Autodesk Inventor part; units mm, degrees
(part 2 of 2)
sketch "Sketch29" plane through (0, 0, -31) normal (0, 0, -1) x (-1, 0, 0)
  line L0 (66.4684, -62.625) -> (66.4684, -59.625) projected
  line L1 (76.0516, -62.625) -> (66.4684, -62.625) projected
  line L2 (76.0516, -59.625) -> (76.0516, -62.625) projected
  line L3 (76.0516, -59.625) -> (66.4684, -59.625) projected
  line L4 (86.26, -59.625) -> (86.26, -56.625) projected
  line L5 (86.26, -56.625) -> (-49.26, -56.625) projected
  arc A0 (-54.26, -51.625) -> (-49.26, -56.625) centre (-49.26, -51.625) ccw projected
  line L6 (-54.26, -51.625) -> (-54.26, 34.625) projected
  line L7 (-54.26, 34.625) -> (-57.26, 34.625) projected
  line L8 (-57.26, 34.625) -> (-57.26, -51.625) projected
  arc A1 (-57.26, -51.625) -> (-49.26, -59.625) centre (-49.26, -51.625) ccw projected
  line L9 (-49.26, -59.625) -> (86.26, -59.625) projected
  line L10 (76.26, -60.625) -> (66.26, -60.625)
  line L11 (66.26, -60.625) -> (66.26, -52.625)
  line L12 (66.26, -52.625) -> (76.26, -52.625)
  line L13 (76.26, -52.625) -> (76.26, -60.625)
  line L14 (50.26, -56.625) -> (86.26, -56.625) projected
  line L15 (76.26, -60.625) -> (66.26, -52.625) construction
  line L16 (66.26, -60.625) -> (76.26, -52.625) construction
  point P0 (0, 0)
  point P1 (71.26, -56.625)
  point P2 (66.26, -56.625)
  point P3 (76.26, -56.625)
  dimension "d214" = 10
  dimension "d215" = 8
  constraints: 12 end point, 2 midpoint, 2 parallel, 1 horizontal, 1 perpendicular, 1 point on line
  measures "d214" distance of L11.end L12.end
  measures "d215" distance of L10.end L11.end
extrude "Extrusion21" add sketch "Sketch29" against normal blind 10 contours L11 L12 L13 L5
sketch "Sketch30" plane through (0, 0, -31) normal (0, 0, -1) x (-1, 0, 0)
  line L0 (86.26, -59.625) -> (86.26, -56.625) projected
  line L1 (86.26, -56.625) -> (76.26, -56.625) projected
  line L2 (76.26, -56.625) -> (76.26, -52.625) projected
  line L3 (76.26, -52.625) -> (66.26, -52.625) projected
  line L4 (66.26, -52.625) -> (66.26, -56.625) projected
  line L5 (66.26, -56.625) -> (-49.26, -56.625) projected
  arc A0 (-54.26, -51.625) -> (-49.26, -56.625) centre (-49.26, -51.625) ccw projected
  line L6 (-54.26, -51.625) -> (-54.26, 34.625) projected
  line L7 (-54.26, 34.625) -> (-57.26, 34.625) projected
  line L8 (-57.26, 34.625) -> (-57.26, -51.625) projected
  arc A1 (-57.26, -51.625) -> (-49.26, -59.625) centre (-49.26, -51.625) ccw projected
  line L9 (-49.26, -59.625) -> (86.26, -59.625) projected
  line L10 (66.26, -56.625) -> (76.26, -56.625)
  line L11 (66.26, -56.625) -> (76.26, -56.625) projected
  line L12 (68.46, -56.625) -> (74.06, -56.625)
  line L13 (74.06, -56.625) -> (74.06, -54.025)
  line L14 (74.06, -54.025) -> (68.46, -54.025)
  line L15 (68.46, -54.025) -> (68.46, -56.625)
  line L16 (76.26, -52.625) -> (66.26, -52.625) projected
  point P0 (0, 0)
  point P1 (71.26, -54.025)
  point P2 (71.26, -52.625)
  point P3 (71.26, -52.625)
  dimension "d218" = 5.6
  dimension "d219" = 2.6
  constraints: 10 end point, 3 midpoint, 2 horizontal, 2 parallel, 1 perpendicular, 1 point on line, 1 vertical alignment
  measures "d218" distance of L14.end L13.end
  measures "d219" distance of L13.end L12.end
extrude "Extrusion22" cut sketch "Sketch30" against normal blind 7 contours L10 L15 L14 L13
chamfer "Chamfer9" distance 2 angle 45 2 edges at (-71.26, -56.625, -21) (-71.26, -52.625, -21)
fillet "Fillet6" radius 3 4 edges at (-76.26, -56.625, -26) (-76.26, -56.625, -20.0001) (-66.26, -56.625, -26) (-66.26, -56.625, -20.0001)
sketch "Sketch31" plane through (0, 0, -31) normal (0, 0, -1) x (-1, 0, 0)
  line L0 (74.06, -56.625) -> (68.46, -56.625) projected
  line L1 (68.46, -56.625) -> (68.46, -54.025) projected
  line L2 (68.46, -54.025) -> (74.06, -54.025) projected
  line L3 (74.06, -54.025) -> (74.06, -56.625) projected
  line L4 (86.26, -59.625) -> (86.26, -56.625) projected
  line L5 (86.26, -56.625) -> (79.26, -56.625) projected
  arc A0 (76.26, -53.625) -> (79.26, -56.625) centre (79.26, -53.625) ccw projected
  line L6 (76.26, -53.625) -> (76.26, -52.625) projected
  line L7 (76.26, -52.625) -> (66.26, -52.625) projected
  line L8 (66.26, -52.625) -> (66.26, -53.625) projected
  arc A1 (63.26, -56.625) -> (66.26, -53.625) centre (63.26, -53.625) ccw projected
  line L9 (63.26, -56.625) -> (-49.26, -56.625) projected
  arc A2 (-54.26, -51.625) -> (-49.26, -56.625) centre (-49.26, -51.625) ccw projected
  line L10 (-54.26, -51.625) -> (-54.26, 34.625) projected
  line L11 (-54.26, 34.625) -> (-57.26, 34.625) projected
  line L12 (-57.26, 34.625) -> (-57.26, -51.625) projected
  arc A3 (-57.26, -51.625) -> (-49.26, -59.625) centre (-49.26, -51.625) ccw projected
  line L13 (-49.26, -59.625) -> (86.26, -59.625) projected
  line L14 (-57.26, -23.1666) -> (-60.26, -23.1666) projected
  line L15 (-57.26, -23.1666) -> (-57.26, -13.5834) projected
  line L16 (-60.26, -13.5834) -> (-57.26, -13.5834) projected
  line L17 (-60.26, -23.1666) -> (-60.26, -13.5834) projected
  line L18 (-58.26, -23.375) -> (-50.26, -23.375)
  line L19 (-50.26, -23.375) -> (-50.26, -13.375)
  line L20 (-50.26, -13.375) -> (-58.26, -13.375)
  line L21 (-58.26, -13.375) -> (-58.26, -23.375)
  line L22 (-54.26, 55.625) -> (-54.26, -51.625) projected
  line L23 (-58.26, -23.375) -> (-50.26, -13.375) construction
  line L24 (-50.26, -23.375) -> (-58.26, -13.375) construction
  point P0 (0, 0)
  point P1 (-54.26, -18.375)
  point P2 (-54.26, -13.375)
  point P3 (-54.26, -23.375)
  dimension "d226" = 8
  dimension "d227" = 10
  constraints: 12 end point, 2 midpoint, 2 parallel, 1 horizontal, 1 perpendicular, 1 point on line
  measures "d226" distance of L20.end L19.end
  measures "d227" distance of L19.end L18.end
extrude "Extrusion23" add sketch "Sketch31" against normal blind 10 contours L10 L20 L19 L18
sketch "Sketch26" plane through (57.26, -51.625, -31) normal (1, 0, 0) x (0, 0, -1)
  arc A0 (-4, 38.25) -> (-4, 28.25) centre (-4, 33.25) ccw projected
  point P0 (-31, 51.625)
hole "Hole6" at (57.26, -18.375, -27) direction (-1, 0, 0) diameter 3.4 depth 8 clearance for "Socket Head Cap Screw" size "M3" standard "Ansi Metric M Profile"
sketch "Sketch27" plane through (-86.26, -59.625, -31) normal (0, -1, 0) x (1, 0, 0)
  arc A0 (20, 4) -> (10, 4) centre (15, 4) ccw projected
  point P0 (86.26, 31)
hole "Hole7" at (-71.26, -59.625, -27) direction (0, 1, 0) diameter 3.4 depth 8 clearance for "Socket Head Cap Screw" size "M3" standard "Ansi Metric M Profile"
sketch "Sketch32" plane through (0, 0, -31) normal (0, 0, -1) x (-1, 0, 0)
  line L0 (74.06, -56.625) -> (68.46, -56.625) projected
  line L1 (68.46, -56.625) -> (68.46, -54.025) projected
  line L2 (68.46, -54.025) -> (74.06, -54.025) projected
  line L3 (74.06, -54.025) -> (74.06, -56.625) projected
  line L4 (86.26, -59.625) -> (86.26, -56.625) projected
  line L5 (86.26, -56.625) -> (79.26, -56.625) projected
  arc A0 (76.26, -53.625) -> (79.26, -56.625) centre (79.26, -53.625) ccw projected
  line L6 (76.26, -53.625) -> (76.26, -52.625) projected
  line L7 (76.26, -52.625) -> (66.26, -52.625) projected
  line L8 (66.26, -52.625) -> (66.26, -53.625) projected
  arc A1 (63.26, -56.625) -> (66.26, -53.625) centre (63.26, -53.625) ccw projected
  line L9 (63.26, -56.625) -> (-49.26, -56.625) projected
  arc A2 (-54.26, -51.625) -> (-49.26, -56.625) centre (-49.26, -51.625) ccw projected
  line L10 (-54.26, -51.625) -> (-54.26, -23.375) projected
  line L11 (-54.26, -23.375) -> (-50.26, -23.375) projected
  line L12 (-50.26, -23.375) -> (-50.26, -13.375) projected
  line L13 (-50.26, -13.375) -> (-54.26, -13.375) projected
  line L14 (-54.26, -13.375) -> (-54.26, 34.625) projected
  line L15 (-54.26, 34.625) -> (-57.26, 34.625) projected
  line L16 (-57.26, 34.625) -> (-57.26, -51.625) projected
  arc A3 (-57.26, -51.625) -> (-49.26, -59.625) centre (-49.26, -51.625) ccw projected
  line L17 (-49.26, -59.625) -> (86.26, -59.625) projected
  line L18 (-54.26, -51.625) -> (-54.26, -23.375) projected
  line L19 (-54.26, -13.375) -> (-54.26, -23.375)
  line L20 (-56.86, -21.175) -> (-51.66, -21.175)
  line L21 (-51.66, -21.175) -> (-51.66, -15.575)
  line L22 (-51.66, -15.575) -> (-56.86, -15.575)
  line L23 (-56.86, -15.575) -> (-56.86, -21.175)
  line L24 (-56.86, -21.175) -> (-51.66, -15.575) construction
  line L25 (-51.66, -21.175) -> (-56.86, -15.575) construction
  point P0 (0, 0)
  point P1 (-54.26, -18.375)
  point P2 (-54.26, -15.575)
  point P3 (-54.26, -21.175)
  dimension "d238" = 5.2
  dimension "d239" = 5.6
  constraints: 14 end point, 3 midpoint, 2 parallel, 1 horizontal, 1 perpendicular, 1 vertical
  measures "d238" distance of L22.end L21.end
  measures "d239" distance of L21.end L20.end
extrude "Extrusion24" cut sketch "Sketch32" against normal blind 7.5 contours L22 L21 L20 L19
chamfer "Chamfer10" distance 2 angle 45 2 edges at (50.26, -18.375, -21) (54.26, -18.375, -21)
fillet "Fillet7" radius 4 4 edges at (54.26, -23.375, -20.0001) (54.26, -23.375, -26) (54.26, -13.375, -20.0001) (54.26, -13.375, -26)
sketch "Sketch33" plane through (-86.26, -62.625, 5.75) normal (0, -1, 0) x (1, 0, 0)
  line L0 (115.9766, -20.7763) -> (-67.1269, -20.7763) construction
  line L1 (-67.1269, -20.7763) -> (-67.1269, -9.2572) construction
  line L2 (-67.1269, -9.2572) -> (115.9766, -9.2572) construction
  line L3 (115.9766, -9.2572) -> (115.9766, -20.7763) construction
  line L4 (115.1682, -20.6377) -> (111.0565, -20.6377)
  spline S0 degree 2 poles (111.0565, -20.6377) (109.7168, -20.6377) (108.377, -19.3595) (108.377, -18.1815) knots 0 0 0 1 2 2 2
  spline S1 degree 2 poles (108.377, -18.1815) (108.377, -16.9649) (109.8323, -15.6021) (111.326, -15.6021) knots 0 0 0 1 2 2 2
  line L5 (111.326, -15.6021) -> (112.6811, -15.6021)
  line L6 (112.6811, -15.6021) -> (112.6811, -12.6377)
  line L7 (112.6811, -12.6377) -> (115.1682, -12.6377)
  line L8 (115.1682, -12.6377) -> (115.1682, -20.6377)
  line L9 (112.6811, -17.2267) -> (112.0806, -17.2267)
  spline S2 degree 2 poles (112.0806, -17.2267) (111.3645, -17.2267) (110.787, -17.7272) (110.787, -18.1122) knots 0 0 0 1 2 2 2
  spline S3 degree 2 poles (110.787, -18.1122) (110.787, -18.4895) (111.2875, -19.0131) (111.9805, -19.0131) knots 0 0 0 1 2 2 2
  line L10 (111.9805, -19.0131) -> (112.6811, -19.0131)
  line L11 (112.6811, -19.0131) -> (112.6811, -17.2267)
  line L12 (107.0835, -20.6377) -> (100.4617, -20.6377)
  line L13 (100.4617, -20.6377) -> (100.4617, -18.9284)
  line L14 (100.4617, -18.9284) -> (104.6041, -18.9284)
  line L15 (104.6041, -18.9284) -> (104.6041, -17.6579)
  line L16 (104.6041, -17.6579) -> (100.762, -17.6579)
  line L17 (100.762, -17.6579) -> (100.762, -16.0256)
  line L18 (100.762, -16.0256) -> (104.6041, -16.0256)
  line L19 (104.6041, -16.0256) -> (104.6041, -14.4471)
  line L20 (104.6041, -14.4471) -> (100.3385, -14.4471)
  line L21 (100.3385, -14.4471) -> (100.3385, -12.6377)
  line L22 (100.3385, -12.6377) -> (107.0835, -12.6377)
  line L23 (107.0835, -12.6377) -> (107.0835, -20.6377)
  line L24 (99.0142, -20.6377) -> (94.9025, -20.6377)
  spline S4 degree 2 poles (94.9025, -20.6377) (93.5628, -20.6377) (92.223, -19.3595) (92.223, -18.1815) knots 0 0 0 1 2 2 2
  spline S5 degree 2 poles (92.223, -18.1815) (92.223, -16.9649) (93.6783, -15.6021) (95.172, -15.6021) knots 0 0 0 1 2 2 2
  line L25 (95.172, -15.6021) -> (96.5271, -15.6021)
  line L26 (96.5271, -15.6021) -> (96.5271, -12.6377)
  line L27 (96.5271, -12.6377) -> (99.0142, -12.6377)
  line L28 (99.0142, -12.6377) -> (99.0142, -20.6377)
  line L29 (96.5271, -17.2267) -> (95.9266, -17.2267)
  spline S6 degree 2 poles (95.9266, -17.2267) (95.2105, -17.2267) (94.633, -17.7272) (94.633, -18.1122) knots 0 0 0 1 2 2 2
  spline S7 degree 2 poles (94.633, -18.1122) (94.633, -18.4895) (95.1335, -19.0131) (95.8265, -19.0131) knots 0 0 0 1 2 2 2
  line L30 (95.8265, -19.0131) -> (96.5271, -19.0131)
  line L31 (96.5271, -19.0131) -> (96.5271, -17.2267)
  line L32 (81.8746, -15.9101) -> (79.711, -15.2556)
  spline S8 degree 2 poles (79.711, -15.2556) (79.9266, -14.347) (80.8659, -13.1228) (82.2596, -12.4991) (83.3298, -12.4991) knots 0 0 0 1 2 3 3 3
  spline S9 degree 2 poles (83.3298, -12.4991) (84.6388, -12.4991) (86.2865, -13.2614) (87.4877, -15.1709) (87.4877, -16.6569) knots 0 0 0 1 2 3 3 3
  spline S10 degree 2 poles (87.4877, -16.6569) (87.4877, -18.6435) (85.378, -20.7763) (83.4453, -20.7763) knots 0 0 0 1 2 2 2
  spline S11 degree 2 poles (83.4453, -20.7763) (81.9362, -20.7763) (80.2115, -19.552) (79.788, -18.2893) knots 0 0 0 1 2 2 2
  line L33 (79.788, -18.2893) -> (81.9747, -17.8042)
  spline S12 degree 2 poles (81.9747, -17.8042) (82.0902, -18.1661) (82.2134, -18.3355) knots 0 0 0 1 1 1
  spline S13 degree 2 poles (82.2134, -18.3355) (82.4213, -18.6204) (83.0219, -18.9284) (83.3914, -18.9284) knots 0 0 0 1 2 2 2
  spline S14 degree 2 poles (83.3914, -18.9284) (84.223, -18.9284) (84.6696, -18.2508) knots 0 0 0 1 1 1
  spline S15 degree 2 poles (84.6696, -18.2508) (85.0084, -17.7503) (85.0084, -16.6723) knots 0 0 0 1 1 1
  spline S16 degree 2 poles (85.0084, -16.6723) (85.0084, -15.3403) (84.1999, -14.3547) (83.4684, -14.3547) knots 0 0 0 1 2 2 2
  spline S17 degree 2 poles (83.4684, -14.3547) (82.7601, -14.3547) (82.0363, -15.1478) (81.8746, -15.9101) knots 0 0 0 1 2 2 2
  spline S18 degree 2 poles (78.8101, -16.6338) (78.8101, -18.5896) (76.6234, -20.7763) (74.6754, -20.7763) knots 0 0 0 1 2 2 2
  spline S19 degree 2 poles (74.6754, -20.7763) (72.6811, -20.7763) (70.5175, -18.6281) (70.5175, -16.6954) knots 0 0 0 1 2 2 2
  spline S20 degree 2 poles (70.5175, -16.6954) (70.5175, -15.2941) (71.4646, -13.5001) (73.2509, -12.4991) (74.583, -12.4991) knots 0 0 0 1 2 3 3 3
  spline S21 degree 2 poles (74.583, -12.4991) (75.9304, -12.4991) (77.7091, -13.3615) (78.8101, -15.2325) (78.8101, -16.6338) knots 0 0 0 1 2 3 3 3
  spline S22 degree 2 poles (76.3385, -16.6184) (76.3385, -15.4096) (75.4376, -14.347) (74.66, -14.347) knots 0 0 0 1 2 2 2
  spline S23 degree 2 poles (74.66, -14.347) (73.8669, -14.347) (72.9891, -15.3865) (72.9891, -16.7262) knots 0 0 0 1 2 2 2
  spline S24 degree 2 poles (72.9891, -16.7262) (72.9891, -17.8581) (73.8977, -18.9053) (74.6831, -18.9053) knots 0 0 0 1 2 2 2
  spline S25 degree 2 poles (74.6831, -18.9053) (75.4299, -18.9053) (76.3385, -17.8427) (76.3385, -16.6184) knots 0 0 0 1 2 2 2
  line L34 (69.147, -12.6377) -> (69.147, -20.6377)
  line L35 (69.147, -20.6377) -> (65.0276, -20.6377)
  spline S26 degree 2 poles (65.0276, -20.6377) (63.8881, -20.6377) (62.6715, -20.245) (61.9323, -19.1824) (61.9323, -18.4202) knots 0 0 0 1 2 3 3 3
  spline S27 degree 2 poles (61.9323, -18.4202) (61.9323, -17.7503) (62.5021, -16.7878) (62.9949, -16.4876) knots 0 0 0 1 2 2 2
  spline S28 degree 2 poles (62.9949, -16.4876) (63.3106, -16.2951) (63.865, -16.1719) knots 0 0 0 1 1 1
  spline S29 degree 2 poles (63.865, -16.1719) (63.4261, -16.0256) (63.2182, -15.8793) knots 0 0 0 1 1 1
  spline S30 degree 2 poles (63.2182, -15.8793) (63.0873, -15.7792) (62.5714, -15.1324) (62.479, -14.9553) knots 0 0 0 1 2 2 2
  line L36 (62.479, -14.9553) -> (61.2856, -12.6377)
  line L37 (61.2856, -12.6377) -> (64.0806, -12.6377)
  line L38 (64.0806, -12.6377) -> (65.3972, -15.0862)
  spline S31 degree 2 poles (65.3972, -15.0862) (65.6436, -15.5559) (65.8361, -15.7022) knots 0 0 0 1 1 1
  spline S32 degree 2 poles (65.8361, -15.7022) (66.1056, -15.887) (66.4444, -15.887) knots 0 0 0 1 1 1
  line L39 (66.4444, -15.887) -> (66.66, -15.887)
  line L40 (66.66, -15.887) -> (66.66, -12.6377)
  line L41 (66.66, -12.6377) -> (69.147, -12.6377)
  line L42 (66.66, -17.3961) -> (65.6205, -17.3961)
  spline S33 degree 2 poles (65.6205, -17.3961) (65.4588, -17.3961) (64.9737, -17.5039) knots 0 0 0 1 1 1
  spline S34 degree 2 poles (64.9737, -17.5039) (64.7273, -17.5578) (64.4194, -17.9582) (64.4194, -18.22) knots 0 0 0 1 2 2 2
  spline S35 degree 2 poles (64.4194, -18.22) (64.4194, -18.605) (64.9044, -19.0208) (65.582, -19.0208) knots 0 0 0 1 2 2 2
  line L43 (65.582, -19.0208) -> (66.66, -19.0208)
  line L44 (66.66, -19.0208) -> (66.66, -17.3961)
  line L45 (60.4925, -20.6377) -> (56.3809, -20.6377)
  spline S36 degree 2 poles (56.3809, -20.6377) (55.0411, -20.6377) (53.7014, -19.3595) (53.7014, -18.1815) knots 0 0 0 1 2 2 2
  spline S37 degree 2 poles (53.7014, -18.1815) (53.7014, -16.9649) (55.1566, -15.6021) (56.6503, -15.6021) knots 0 0 0 1 2 2 2
  line L46 (56.6503, -15.6021) -> (58.0055, -15.6021)
  line L47 (58.0055, -15.6021) -> (58.0055, -12.6377)
  line L48 (58.0055, -12.6377) -> (60.4925, -12.6377)
  line L49 (60.4925, -12.6377) -> (60.4925, -20.6377)
  line L50 (58.0055, -17.2267) -> (57.4049, -17.2267)
  spline S38 degree 2 poles (57.4049, -17.2267) (56.6888, -17.2267) (56.1114, -17.7272) (56.1114, -18.1122) knots 0 0 0 1 2 2 2
  spline S39 degree 2 poles (56.1114, -18.1122) (56.1114, -18.4895) (56.6118, -19.0131) (57.3048, -19.0131) knots 0 0 0 1 2 2 2
  line L51 (57.3048, -19.0131) -> (58.0055, -19.0131)
  line L52 (58.0055, -19.0131) -> (58.0055, -17.2267)
  line L53 (52.5464, -14.8629) -> (50.1749, -14.8629)
  line L54 (50.1749, -14.8629) -> (50.1749, -12.6377)
  line L55 (50.1749, -12.6377) -> (52.5464, -12.6377)
  line L56 (52.5464, -12.6377) -> (52.5464, -14.8629)
  line L57 (45.7476, -20.6377) -> (43.1604, -20.6377)
  line L58 (43.1604, -20.6377) -> (41.351, -14.8783)
  line L59 (41.351, -14.8783) -> (39.5801, -20.6377)
  line L60 (39.5801, -20.6377) -> (37.07, -20.6377)
  line L61 (37.07, -20.6377) -> (40.0421, -12.6377)
  line L62 (40.0421, -12.6377) -> (42.7216, -12.6377)
  line L63 (42.7216, -12.6377) -> (45.7476, -20.6377)
  line L64 (30.1094, -12.6377) -> (36.7774, -12.6377)
  spline S40 degree 2 poles (36.7774, -12.6377) (36.6619, -13.6233) (35.4992, -15.3634) (33.8977, -16.5491) knots 0 0 0 1 2 2 2
  spline S41 degree 2 poles (33.8977, -16.5491) (32.9275, -17.2729) (32.3809, -18.0275) (32.3809, -18.3663) knots 0 0 0 1 2 2 2
  spline S42 degree 2 poles (32.3809, -18.3663) (32.3809, -18.7359) (32.9198, -19.2517) (33.3279, -19.2517) knots 0 0 0 1 2 2 2
  spline S43 degree 2 poles (33.3279, -19.2517) (33.7591, -19.2517) (34.2981, -18.7205) (34.3905, -18.0429) knots 0 0 0 1 2 2 2
  line L65 (34.3905, -18.0429) -> (36.6157, -18.22)
  spline S44 degree 2 poles (36.6157, -18.22) (36.4848, -19.1594) (35.7841, -20.2142) (34.5137, -20.7763) (33.3895, -20.7763) knots 0 0 0 1 2 3 3 3
  spline S45 degree 2 poles (33.3895, -20.7763) (32.2192, -20.7763) (30.9102, -20.2373) (30.1633, -19.1363) (30.1633, -18.4433) knots 0 0 0 1 2 3 3 3
  spline S46 degree 2 poles (30.1633, -18.4433) (30.1633, -17.7118) (31.018, -16.3798) (32.1499, -15.579) knots 0 0 0 1 2 2 2
  spline S47 degree 2 poles (32.1499, -15.579) (32.8197, -15.117) (33.274, -14.7474) (33.582, -14.4471) knots 0 0 0 1 2 2 2
  line L66 (33.582, -14.4471) -> (30.1094, -14.4471)
  line L67 (30.1094, -14.4471) -> (30.1094, -12.6377)
  point P0 (86.26, -5.75)
  constraints: 2 other
extrude "Extrusion25" cut sketch "Sketch33" against normal blind 0.5
body "Solid1"
